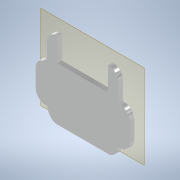
# Autodesk Inventor part: bottom-bracket
Saved by Autodesk Inventor 2020 (Build 240168000, 168)
## iProperties
Created: 2019-11-08
Part Number: bottom-bracket
Material: Aluminum 6061
Document SubType Name: Modeling
Designer: Hymowitz
Density: 2.7 g/cm^3
Sheet Metal Width: 0.000 in
Sheet Metal Length: 0.000 in
Sheet Metal Area: 0.000 in^2
Appearance: Aluminum - Flat
Sheet Metal Rule: Default
Author: Hymowitz
## iProperties of the stored document _3DPrint.ipt
Created: 2019-11-25
Part Number: _3DPrint
Material: Generic
Document SubType Name: Modeling
Designer: Hymowitz
Density: 1 g/cm^3
Appearance: Default
Author: Hymowitz
Autodesk Inventor part; units mm, degrees
ref_plane "YZ Plane" through (0, 0, 0) normal (1, 0, 0) x (0, 1, 0)
ref_plane "XZ Plane" through (0, 0, 0) normal (0, 1, 0) x (-1, 0, 0)
ref_plane "XY Plane" through (0, 0, 0) normal (0, 0, 1) x (1, 0, 0)
ref_plane "Work Plane1" through (3.6062, 5.0251, 0) normal (0, 0, 1) x (1, 0, 0)
sketch "Sketch1" plane through (3.6062, 5.0251, 0) normal (0, 0, 1) x (1, 0, 0)
  line L0 (-59.3453, 14.0249) -> (-60.5022, 14.0249)
  ellipse E0 centre (-52.8822, 15.9436) end of major axis (-52.8822, 6.6041) minor radius 6.604 (-59.3453, 14.0249) -> (-52.8822, 6.6041) ccw
  line L1 (-52.8822, 6.6041) -> (-17.8302, 6.6041)
  ellipse E1 centre (-17.8302, 15.9436) end of major axis (-17.8302, 25.2831) minor radius 6.604 (-17.8302, 6.6041) -> (-11.367, 14.0249) ccw
  line L2 (-10.2102, 14.0249) -> (-11.367, 14.0249)
  arc A0 (-10.2102, 14.0249) -> (-3.6062, 20.6289) centre (-10.2102, 20.6289) ccw
  line L3 (-3.6062, 20.6289) -> (-3.6062, 32.8209)
  arc A1 (-3.6062, 32.8209) -> (-10.2102, 39.4249) centre (-10.2102, 32.8209) ccw
  line L4 (-11.2262, 39.4249) -> (-10.2102, 39.4249)
  line L5 (-11.2262, 51.8709) -> (-11.2262, 39.4249)
  arc A2 (-11.2262, 51.8709) -> (-17.8302, 58.4749) centre (-17.8302, 51.8709) ccw
  line L6 (-17.8302, 58.4749) -> (-52.8822, 58.4749)
  arc A3 (-52.8822, 58.4749) -> (-59.4862, 51.8709) centre (-52.8822, 51.8709) ccw
  line L7 (-59.4862, 39.4249) -> (-59.4862, 51.8709)
  line L8 (-60.5022, 39.4249) -> (-59.4862, 39.4249)
  arc A4 (-60.5022, 39.4249) -> (-67.1062, 32.8209) centre (-60.5022, 32.8209) ccw
  line L9 (-67.1062, 20.6289) -> (-67.1062, 32.8209)
  arc A5 (-67.1062, 20.6289) -> (-60.5022, 14.0249) centre (-60.5022, 20.6289) ccw
  line L10 (-52.8822, 6.6041) -> (-17.8302, 6.6041)
  point P0 (-3.6062, -5.0251)
extrude "Plate1" add sketch "Sketch1" along normal blind 3.048
sketch "Sketch2" plane through (3.6062, 5.0251, 3.048) normal (0, 0, 1) x (1, 0, 0)
  line L0 (-19.2272, 69.2699) -> (-19.2272, 51.2359) projected
  line L1 (-42.2142, 43.5397) -> (-28.4982, 43.5397) projected
  line L2 (-51.4852, 51.2359) -> (-51.4852, 69.2699) projected
  line L3 (-19.2272, 58.5208) -> (-19.2272, 43.5397)
  line L4 (-19.2272, 43.5397) -> (-51.4852, 43.5397)
  line L5 (-51.4852, 43.5397) -> (-51.4852, 64.3147)
  line L6 (-52.4852, 58.4749) -> (-52.4852, 42.5397)
  line L7 (-52.4852, 42.5397) -> (-18.2272, 42.5397)
  line L8 (-18.2272, 42.5397) -> (-18.2272, 58.5208)
  line L9 (-52.8822, 58.4749) -> (-17.8302, 58.4749) projected
  point P0 (0, 0)
  point P1 (-18.2272, 58.4749)
  dimension "d2" = 1
  constraints: 12 end point, 3 point on line, 1 vertical, 2 other
  measures "d2" distance between parallel lines of L4 L7
extrude "Extrusion2" cut sketch "Sketch2" against normal through all
sketch "Sketch4" plane through (3.6062, 5.0251, 3.048) normal (0, 0, 1) x (1, 0, 0)
  line L0 (-12.8862, 21.4549) -> (-12.8862, 17.4549) projected
  line L1 (-9.0098, 35.2125) -> (-13.2052, 35.2125)
  line L2 (-13.2052, 35.2125) -> (-13.2052, 18.2304)
  line L3 (-13.2052, 18.2304) -> (-12.8862, 18.2304)
  line L4 (-9.0098, 16.8588) -> (-9.0098, 35.2125)
  line L5 (-9.0098, 35.2125) -> (-13.2052, 18.2304) construction
  line L6 (-13.2052, 35.2125) -> (-9.0098, 16.8588) construction
  line L7 (-12.8862, 21.4549) -> (-12.8862, 17.4549) projected
  line L8 (-3.6062, 30.2174) -> (-8.2582, 30.2174)
  line L9 (-12.8862, 17.9549) -> (-3.6562, 17.9549)
  line L10 (-12.8862, 21.4549) -> (-12.8862, 17.4549) projected
  line L11 (-13.2052, 18.2304) -> (-12.8862, 18.2304)
  line L12 (-9.0098, 16.8588) -> (-9.0098, 12.9511)
  line L13 (-9.0098, 12.9511) -> (-13.2052, 12.9511)
  line L14 (-13.2052, 12.9511) -> (-13.2052, 18.2304)
  point P0 (-3.6062, -5.0251)
  point P1 (-11.1889, 26.3919)
  point P2 (-11.1075, 26.7215)
  dimension "d18" = 4.1954
  dimension "d23" = 4.9951
  dimension "d24" = 0.3191
  dimension "d25" = 5.0038
  constraints: 24 end point, 4 horizontal, 4 parallel, 3 point on line, 2 perpendicular, 1 midpoint, 5 other
  measures "d18" distance between parallel lines of L4 L2
  measures "d23" distance between parallel lines of L8 L1
  measures "d24" distance between parallel lines of L0 L2
  measures "d25" distance between parallel lines of L13 L9
extrude "Extrusion3" cut sketch "Sketch4" against normal blind 2
sketch "Sketch5" plane through (3.6062, 5.0251, 3.048) normal (0, 0, 1) x (1, 0, 0)
  line L0 (-52.4852, 42.5397) -> (-52.4852, 58.4749) projected
  line L1 (-52.8822, 58.4749) -> (-52.4852, 58.4749) projected
  arc A0 (-52.8822, 58.4749) -> (-59.4862, 51.8709) centre (-52.8822, 51.8709) ccw projected
  line L2 (-59.4862, 39.4249) -> (-59.4862, 51.8709) projected
  line L3 (-60.5022, 39.4249) -> (-59.4862, 39.4249) projected
  arc A1 (-60.5022, 39.4249) -> (-67.1062, 32.8209) centre (-60.5022, 32.8209) ccw projected
  line L4 (-67.1062, 20.6289) -> (-67.1062, 32.8209) projected
  arc A2 (-67.1062, 20.6289) -> (-60.5022, 14.0249) centre (-60.5022, 20.6289) ccw projected
  line L5 (-59.3453, 14.0249) -> (-60.5022, 14.0249) projected
  ellipse E0 centre (-52.8822, 15.9436) end of major axis (-52.8822, 6.6041) minor radius 6.604 (-59.3453, 14.0249) -> (-52.8822, 6.6041) ccw projected
  line L6 (-17.8302, 6.6041) -> (-52.8822, 6.6041) projected
  ellipse E1 centre (-17.8302, 15.9436) end of major axis (-17.8302, 25.2831) minor radius 6.604 (-17.8302, 6.6041) -> (-11.5743, 12.9511) ccw projected
  arc A3 (-9.0098, 14.1349) -> (-3.6062, 20.6289) centre (-10.2102, 20.6289) ccw projected
  line L7 (-3.6062, 32.8209) -> (-3.6062, 20.6289) projected
  arc A4 (-3.6062, 32.8209) -> (-10.2102, 39.4249) centre (-10.2102, 32.8209) ccw projected
  line L8 (-11.2262, 39.4249) -> (-10.2102, 39.4249) projected
  line L9 (-11.2262, 51.8709) -> (-11.2262, 39.4249) projected
  arc A5 (-11.2262, 51.8709) -> (-17.8302, 58.4749) centre (-17.8302, 51.8709) ccw projected
  line L10 (-18.2272, 58.4749) -> (-17.8302, 58.4749) projected
  line L11 (-18.2272, 58.4749) -> (-18.2272, 42.5397) projected
  line L12 (-18.2272, 42.5397) -> (-52.4852, 42.5397) projected
  line L13 (-13.2052, 12.9511) -> (-13.2052, 35.2125) projected
  line L14 (-44.45, 12.7) -> (-13.2052, 12.7)
  line L15 (-13.2052, 12.7) -> (-13.2052, 26.7215)
  line L16 (-13.2052, 26.7215) -> (-44.45, 26.7215)
  line L17 (-44.45, 26.7215) -> (-44.45, 12.7)
  line L18 (-11.5743, 12.9511) -> (-13.2052, 12.9511) projected
  line L19 (-13.2052, 12.9511) -> (-13.2052, 35.2125) projected
  line L20 (-13.2052, 35.2125) -> (-9.0098, 35.2125) projected
  line L21 (-9.0098, 35.2125) -> (-9.0098, 14.1349) projected
  point P0 (-3.6062, -5.0251)
  point P1 (-13.2052, 18.2304)
  point P2 (-41.0062, 13.5399)
  point P3 (-60.0729, 27.6299)
  dimension "d19" = 14.0215
  dimension "d20" = 31.2448
  constraints: 8 end point, 2 parallel, 1 horizontal, 1 perpendicular, 1 point on line, 4 other
  measures "d19" distance of L16.end L14.start
  measures "d20" distance of L14.start L14.end
extrude "Extrusion4" cut sketch "Sketch5" against normal blind 58.7375 contours L13 L15 L14 L17 L16
sketch "Sketch6" plane through (3.6062, 5.0251, 0) normal (0, 0, -1) x (-1, 0, 0)
  line L0 (13.2052, 12.7) -> (44.45, 12.7) projected
  line L1 (13.2052, 26.7215) -> (44.45, 26.7215) projected
  line L2 (44.45, 12.7) -> (13.2052, 12.7) projected
  line L3 (21.1013, 12.7) -> (21.1013, 26.7215)
  line L4 (15.3165, 12.7) -> (15.3165, 26.7215)
  point P0 (3.6062, -5.0251)
  constraints: 4 end point, 4 point on line, 1 parallel, 1 perpendicular
extrude "Extrusion5" add sketch "Sketch6" against normal blind 1.1906
sketch "Sketch7" plane through (3.6062, 5.0251, 0) normal (0, 0, -1) x (-1, 0, 0)
  line L0 (67.1062, 25.4549) -> (67.1062, 31.8049) projected
  line L1 (67.1062, 31.8049) -> (63.9312, 31.8049) projected
  line L2 (63.9312, 31.8049) -> (63.9312, 25.4549) projected
  line L3 (63.9312, 25.4549) -> (67.1062, 25.4549) projected
  line L4 (57.5812, 31.8049) -> (57.5812, 25.4549) projected
  line L5 (57.5812, 25.4549) -> (60.7562, 25.4549) projected
  line L6 (60.7562, 25.4549) -> (60.7562, 31.8049) projected
  line L7 (60.7562, 31.8049) -> (57.5812, 31.8049) projected
  line L8 (6.4587, 31.8049) -> (6.4587, 25.4549) projected
  line L9 (6.4587, 25.4549) -> (9.3112, 25.4549) projected
  line L10 (9.3112, 25.4549) -> (9.3112, 31.8049) projected
  line L11 (9.3112, 31.8049) -> (6.4587, 31.8049) projected
  line L12 (19.4712, 25.4549) -> (19.4712, 31.8049) projected
  line L13 (19.4712, 31.8049) -> (16.2962, 31.8049) projected
  line L14 (16.2962, 31.8049) -> (16.2962, 25.4549) projected
  line L15 (16.2962, 25.4549) -> (19.4712, 25.4549) projected
  point P0 (3.6062, -5.0251)
extrude "Extrusion6" cut sketch "Sketch7" against normal blind 3.175
sketch "Sketch8" plane through (-60.325, 30.48, 0) normal (-1, 0, 0) x (0, 0, 1)
  circle A0 centre (1.4605, 3.175) radius 0.75 projected
  point P0 (0, -30.48)
extrude "Extrusion7" cut sketch "Sketch8" against normal through all
equation "\"d5\" = Thickness"
equation "\"BendRadius\" = Thickness"
equation "\"BendReliefWidth\" = Thickness"
equation "\"BendReliefDepth\" = 0.5 * Thickness"
equation "\"CornerReliefSize\" = 4 * Thickness"
equation "\"MinimumRemnant\" = 2 * Thickness"
equation "\"TransitionRadius\" = BendRadius"
equation "\"JacobiRadiusSize\" = Thickness"
equation "\"GapSize\" = Thickness"
equation "\"Thickness\" = 3.048"
body "Solid1"
